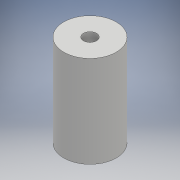
# Autodesk Inventor part: 기본 투상 연습6
Saved by Autodesk Inventor 2018.3 (Build 223284000, 284)
## iProperties
Created: 2019-10-08
Part Number: 기본 투상 연습6
Material: 일반
Document SubType Name: Modeling
Designer: MyTool
Density: 1 g/cm^3
Appearance: 기본값
Author: MyTool
Autodesk Inventor part; units mm, degrees
ref_plane "YZ Plane" through (0, 0, 0) normal (1, 0, 0) x (0, 1, 0)
ref_plane "XZ Plane" through (0, 0, 0) normal (0, 1, 0) x (-1, 0, 0)
ref_plane "XY Plane" through (0, 0, 0) normal (0, 0, 1) x (1, 0, 0)
sketch "스케치2" plane through (0, 0, 0) normal (1, 0, 0) x (0, 1, 0)
  line L0 (0, 0) -> (0, 70)
  line L1 (0, 70) -> (5, 70)
  line L2 (5, 70) -> (20, 70)
  line L3 (20, 70) -> (20, 0)
  line L4 (20, 0) -> (15, 0)
  line L5 (15, 0) -> (15, 25)
  line L6 (15, 25) -> (5, 50)
  line L7 (5, 50) -> (5, 70)
  dimension "d7" = 70
  dimension "d8" = 5
  dimension "d9" = 15
  dimension "d10" = 5
  dimension "d11" = 25
  dimension "d12" = 20
  dimension "d13" = 25
  constraints: 16 end point, 4 perpendicular, 2 vertical, 1 point on line
  measures "d7" distance of L0.start L0.end
  measures "d8" distance of L0.end L1.end
  measures "d9" distance of L1.end L2.end
  measures "d10" distance of L3.end L4.end
  measures "d11" distance of L4.end L5.end
  measures "d12" distance of L6.end L1.end
  measures "d13" vertical distance of L5.end L6.end
revolve "회전2" add sketch "스케치2" angle 360 about axis through (0, 0, 0) along (0, 0, 1)
